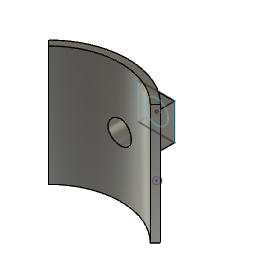
acople_manometro (Autodesk Fusion 360 design; units mm, degrees)
Autodesk Fusion 360 part; units mm, degrees
sketch "Boceto1" plane through (0, 0, 0) normal (0, 0, 1) x (1, 0, 0)
  line L0 (0, 0) -> (23.3345, 23.3345)
  line L1 (0, 0) -> (33, 0) construction
  line L2 (0, 0) -> (-23.3345, 23.3345)
  arc A0 (33, 0) -> (-23.3345, 23.3345) centre (0, 0) ccw
  arc A1 (21.2132, 21.2132) -> (-21.2132, 21.2132) centre (0, 0) ccw
  dimension "d1" = 60
  dimension "d3" = 45
  constraint coincident L0.start L1.start
  constraint horizontal L1
  constraint coincident L0.end A0
  constraint perpendicular L0 L2
  constraint concentric A0 A1
  constraint coincident L2 A1.end
  constraint coincident L0 A1.start
  measures "d1" diameter of A1
  measures "d3" angle of L0 L1
extrude "Extruir1" add sketch "Boceto1" along normal blind 50 contours L0 L2 A0 A1
ref_plane "PlanoDeObra1" through (0, 45, 0) normal (0, 1, 0) x (0, 0, 1)
sketch "Boceto2" plane through (0, 45, 0) normal (0, 1, 0) x (1, 0, 0)
  circle A0 centre (0.0223, -25) radius 4.85
  line L0 (7.5223, -17.5) -> (-7.4777, -17.5)
  line L1 (-7.4777, -17.5) -> (-7.4777, -32.5)
  line L2 (-7.4777, -32.5) -> (7.5223, -32.5)
  line L3 (7.5223, -32.5) -> (7.5223, -17.5)
  line L4 (7.5223, -17.5) -> (-7.4777, -32.5) construction
  line L5 (-7.4777, -17.5) -> (7.5223, -32.5) construction
  point P0 (0.0223, -25)
  dimension "d7" = 9.7
  dimension "d8" = 25
  dimension "d9" = 15
  dimension "d10" = 15
  constraint horizontal L0
  constraint perpendicular L0 L1
  constraint parallel L0 L2
  constraint parallel L1 L3
  constraint coincident L4 P0
  constraint coincident L5 P0
  constraint coincident P0 A0.centre
  measures "d7" diameter of A0
  measures "d8" vertical distance of origin A0.centre
  measures "d9" distance of L1.end L2.end
  measures "d10" distance of L0.end L1.end
extrude "Extruir2" add sketch "Boceto2" against normal blind 14
extrude "Extruir3" cut sketch "Boceto2" against normal blind 31 contours A0
